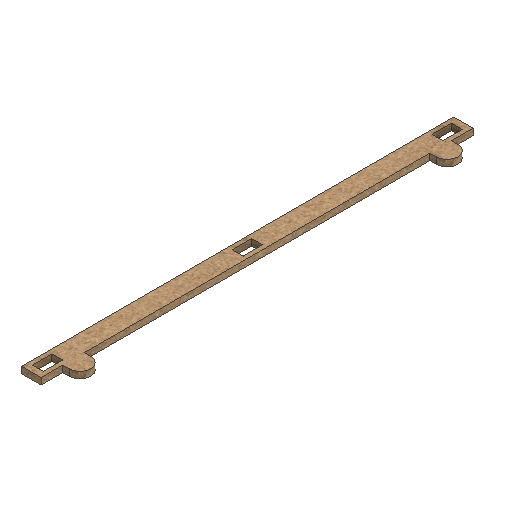
# Autodesk Inventor part: upper_Bar_3
Saved by Autodesk Inventor 2024 (Build 280153000, 153)
## iProperties
Created: 2024-04-09
Part Number: upper_Bar_3
Material: MDF Medium Density Fiberboard
Document SubType Name: Modeling
Designer: USER
Density: 0.8 g/cm^3
Appearance: Cardboard - Corrugated
Mass: 4.3285 g
Surface Area: 51.8333 cm^2
Volume: 5.41062 cm^3
Author: USER
Autodesk Inventor part; units mm, degrees
ref_plane "YZ Plane" through (0, 0, 0) normal (1, 0, 0) x (0, 1, 0)
ref_plane "XZ Plane" through (0, 0, 0) normal (0, 1, 0) x (-1, 0, 0)
ref_plane "XY Plane" through (0, 0, 0) normal (0, 0, 1) x (1, 0, 0)
sketch "草圖1" plane through (0, 0, 0) normal (0, 1, 0) x (-1, 0, 0)
  line L0 (0, 80) -> (9, 80)
  line L1 (9, 80) -> (9, -80)
  line L2 (9, -80) -> (0, -80)
  line L3 (0, -80) -> (0, 80)
  line L4 (7, 4.5) -> (2, 4.5)
  line L5 (2, 4.5) -> (2, -4.5)
  line L6 (2, -4.5) -> (7, -4.5)
  line L7 (7, -4.5) -> (7, 4.5)
  line L8 (9, 80) -> (9, 90)
  line L9 (9, 90) -> (-3, 90)
  line L10 (-8, 85) -> (-8, 85)
  line L11 (-3, 80) -> (0, 80)
  arc A0 (-8, 85) -> (-3, 80) centre (-3, 85) ccw
  arc A1 (-3, 90) -> (-8, 85) centre (-3, 85) ccw
  circle A2 centre (-3, 85) radius 2.5
  line L12 (9, 0) -> (0, 0)
  line L13 (9, -80) -> (9, -90)
  line L14 (9, -90) -> (-3, -90)
  line L15 (-3, -80) -> (0, -80)
  arc A3 (-3, -80) -> (-8, -85) centre (-3, -85) ccw
  arc A4 (-8, -85) -> (-3, -90) centre (-3, -85) ccw
  circle A5 centre (-3, -85) radius 2.5
  line L16 (9, 90) -> (0, 90)
  line L17 (0, 90) -> (0, 100)
  line L18 (0, 100) -> (9, 100)
  line L19 (9, 100) -> (9, 90)
  line L20 (9, -90) -> (0, -90)
  line L21 (0, -90) -> (0, -100)
  line L22 (0, -100) -> (9, -100)
  line L23 (9, -100) -> (9, -90)
  line L24 (7, 97) -> (2, 97)
  line L25 (2, 97) -> (2, 88)
  line L26 (2, 88) -> (7, 88)
  line L27 (7, 88) -> (7, 97)
  line L28 (7, -97) -> (2, -97)
  line L29 (2, -97) -> (2, -88)
  line L30 (2, -88) -> (7, -88)
  line L31 (7, -88) -> (7, -97)
  point P0 (7, 0)
  point P1 (4.5, 4.5)
  point P2 (4.5, 80)
  point P3 (-8, 90)
  point P4 (-8, -90)
  point P5 (-8, -85)
  point P6 (4.5, 97)
  point P7 (4.5, 100)
  point P8 (4.5, -97)
  dimension "d0" = 160
  dimension "d1" = 9
  dimension "d2" = 9
  dimension "d3" = 5
  dimension "d4" = 10
  dimension "d5" = 17
  dimension "d6" = 5
  dimension "d7" = 5
  dimension "d8" = 5
  dimension "d11" = 9
  dimension "d12" = 10
  dimension "d13" = 10
  dimension "d14" = 9
  dimension "d15" = 5
  dimension "d16" = 9
  dimension "d17" = 3
  constraints: 64 end point, 14 symmetric about line, 10 parallel, 8 perpendicular, 8 point on circle, 7 midpoint, 6 centre point, 6 horizontal, 4 tangent, 3 coincident, 3 point on line, 2 vertical alignment, 1 horizontal alignment, 1 vertical, 3 other
  measures "d0" distance of L0.end L1.end
  measures "d1" distance of L0.start L0.end
  measures "d2" distance of L6.end L4.start
  measures "d3" distance of L5.end L6.end
  measures "d4" distance of L0.end L8.end
  measures "d5" distance of L8.end point (-8, 90)
  measures "d6" radius of A0
  measures "d7" radius of A1
  measures "d8" diameter of A2
  measures "d11" distance of L17.end L18.end
  measures "d12" distance of L18.end L8.end
  measures "d13" distance of L22.end L14.start
  measures "d14" distance of L21.end L22.end
  measures "d15" distance of L24.start L24.end
  measures "d16" distance of L26.end L24.start
  measures "d17" vertical distance of L17.end L24.end
extrude "擠出1" add sketch "草圖1" along normal blind 3 contours L11 A0 A1 L9 L25 L26 L27 L8 L0 | L0 L1 L12 L7 L4 L5 L3 | L12 L5 L6 L7 L1 L2 L3 | L9 L27 L24 L25 L17 L18 L19 | L2 L13 L14 L31 L30 L29 A4 A3 L15 | L23 L22 L21 L14 L29 L28 L31 | A2 | A5
